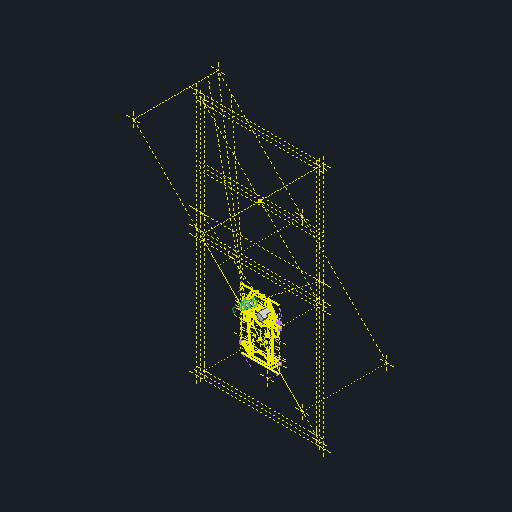
# Autodesk Inventor part: sensormount
Saved by Autodesk Inventor 2023.5 (Build 275446000, 446)
## iProperties
Created: 2025-01-19
Part Number: sensormount
Material: 一般
Document SubType Name: Modeling
Designer: IshiiLabHonda
Density: 1 g/cm^3
Appearance: 既定
Author: IshiiLabHonda
Autodesk Inventor part; units mm, degrees
ref_plane "YZ Plane" through (0, 0, 0) normal (1, 0, 0) x (0, 1, 0)
ref_plane "XZ Plane" through (0, 0, 0) normal (0, 1, 0) x (-1, 0, 0)
ref_plane "XY Plane" through (0, 0, 0) normal (0, 0, 1) x (1, 0, 0)
derived "chassis.ipt"
sketch "スケッチ1" plane through (0, 0, 0) normal (0, 0, 1) x (1, 0, 0)
  line L0 (-90, 90) -> (90, 90) construction
  line L1 (90, 90) -> (90, -90) construction
  line L2 (90, -90) -> (-90, -90) construction
  line L3 (-90, -90) -> (-90, 90) construction
  line L4 (-90, 90) -> (-90, 270) construction
  line L5 (-90, 270) -> (90, 270) construction
  line L6 (90, 270) -> (90, 90) construction
  line L7 (-90, 90) -> (90, -90) construction
  line L8 (90, 90) -> (-90, -90) construction
  line L9 (0, 0) -> (0, 10) construction
  line L10 (0, 0) -> (10, 0) construction
  line L11 (-90, 270) -> (90, 90) construction
  line L12 (-90, 90) -> (90, 270) construction
  line L13 (-96, 276) -> (96, 276) construction
  line L14 (96, 276) -> (96, -96) construction
  line L15 (96, -96) -> (-96, -96) construction
  line L16 (-96, -96) -> (-96, 276) construction
  line L17 (-84, 264) -> (84, 264) construction
  line L18 (84, 264) -> (84, -84) construction
  line L19 (84, -84) -> (-84, -84) construction
  line L20 (-84, -84) -> (-84, 264) construction
  line L21 (-96, 96) -> (96, 96) construction
  line L22 (-96, 84) -> (96, 84) construction
  line L23 (-63.6396, 63.6396) -> (63.6396, 190.9188) construction
  line L24 (63.6396, 190.9188) -> (190.9188, 63.6396) construction
  line L25 (190.9188, 63.6396) -> (63.6396, -63.6396) construction
  line L26 (63.6396, -63.6396) -> (-63.6396, 63.6396) construction
  line L27 (-190.9188, 190.9188) -> (-63.6396, 318.1981) construction
  line L28 (-63.6396, 318.1981) -> (63.6396, 190.9188) construction
  line L29 (-63.6396, 63.6396) -> (-190.9188, 190.9188) construction
  line L30 (-96, 120) -> (96, 120) construction
  line L31 (-96, 186) -> (96, 186) construction
  line L32 (-96, 174) -> (96, 174) construction
  line L33 (-96, 180) -> (96, 180) construction
  point P0 (-63.6396, 318.1981)
  point P1 (-90, 120)
  point P2 (90, 120)
  point P3 (0, 180)
sketch "スケッチ2" plane through (0, 0, 0) normal (0, 0, 1) x (1, 0, 0)
  line L0 (63.6396, 190.9188) -> (190.9188, 63.6396) construction
  line L1 (-63.6396, 318.1981) -> (63.6396, 190.9188) construction
  line L2 (-84, 264) -> (84, 264) construction
  line L3 (-90, 270) -> (90, 270) construction
  line L4 (90, 270) -> (90, 90) construction
  line L5 (-96, 276) -> (96, 276) construction
  line L6 (-90, 90) -> (90, 270) construction
  line L7 (-90, 270) -> (90, 90) construction
  line L8 (-63.6396, 63.6396) -> (63.6396, 190.9188) construction
  line L9 (-96, 120) -> (96, 120) construction
  line L10 (-90, 90) -> (90, 90) construction
  line L11 (-96, 96) -> (96, 96) construction
  line L12 (-96, 84) -> (96, 84) construction
  line L13 (90, -90) -> (-90, -90) construction
  line L14 (0, 0) -> (0, 10) construction
  line L15 (0, 0) -> (10, 0) construction
  line L16 (190.9188, 63.6396) -> (63.6396, -63.6396) construction
  line L17 (63.6396, -63.6396) -> (-63.6396, 63.6396) construction
  line L18 (84, -84) -> (-84, -84) construction
  line L19 (96, -96) -> (-96, -96) construction
  line L20 (-90, 90) -> (-90, 270) construction
  line L21 (-63.6396, 63.6396) -> (-190.9188, 190.9188) construction
  line L22 (-190.9188, 190.9188) -> (-63.6396, 318.1981) construction
  line L23 (96, 276) -> (96, -96) construction
  line L24 (-96, -96) -> (-96, 276) construction
  line L25 (84, 264) -> (84, -84) construction
  line L26 (-84, -84) -> (-84, 264) construction
  line L27 (90, 90) -> (90, -90) construction
  line L28 (-90, 90) -> (90, -90) construction
  line L29 (90, 90) -> (-90, -90) construction
  line L30 (-90, -90) -> (-90, 90) construction
  circle A0 centre (0, 0) radius 16 construction
  circle A1 centre (0, 0) radius 7.5 construction
  line L31 (20, 11.5) -> (28.75, 11.5) construction
  line L32 (28.75, 11.5) -> (28.75, -11.5) construction
  line L33 (28.75, -11.5) -> (20, -11.5) construction
  line L34 (20, -11.5) -> (20, 11.5) construction
  line L35 (20, 11.5) -> (18, 11.5) construction
  line L36 (18, 11.5) -> (18, -11.5) construction
  line L37 (18, -11.5) -> (20, -11.5) construction
  line L38 (18, 1.5) -> (17, 1.5) construction
  line L39 (17, -1.5) -> (18, -1.5) construction
  line L40 (-17, 26) -> (17, 26) construction
  line L41 (17, 26) -> (17, -20) construction
  line L42 (17, -20) -> (-17, -20) construction
  line L43 (-17, -20) -> (-17, 26) construction
  line L44 (-20, 11.5) -> (-18, 11.5) construction
  line L45 (-17, -1.5) -> (-18, -1.5) construction
  line L46 (-20, -11.5) -> (-20, 11.5) construction
  line L47 (-18, 11.5) -> (-18, -11.5) construction
  line L48 (-28.75, -11.5) -> (-20, -11.5) construction
  line L49 (-20, 11.5) -> (-28.75, 11.5) construction
  line L50 (-28.75, 11.5) -> (-28.75, -11.5) construction
  line L51 (-18, -11.5) -> (-20, -11.5) construction
  line L52 (-18, 1.5) -> (-17, 1.5) construction
  line L53 (-14.5, 26) -> (-14.5, -20) construction
  line L54 (14.5, 26) -> (14.5, -20) construction
  line L55 (-10.5, 26) -> (-10.5, 21) construction
  line L56 (-10.5, 21) -> (-14.5, 21) construction
  line L57 (-14.5, 26) -> (-10.5, 21) construction
  line L58 (-10.5, 26) -> (-14.5, 21) construction
  circle A2 centre (-12.5, 23.5) radius 1 construction
  line L59 (10.5, 26) -> (10.5, 21) construction
  line L60 (10.5, 21) -> (14.5, 21) construction
  line L61 (10.5, 26) -> (14.5, 21) construction
  line L62 (10.5, 21) -> (14.5, 26) construction
  circle A3 centre (12.5, 23.5) radius 1 construction
  line L63 (-14.5, -15) -> (-10.5, -15) construction
  line L64 (-10.5, -15) -> (-10.5, -20) construction
  line L65 (10.5, -20) -> (10.5, -15) construction
  line L66 (10.5, -15) -> (14.5, -15) construction
  line L67 (-14.5, -15) -> (-10.5, -20) construction
  line L68 (-10.5, -15) -> (-14.5, -20) construction
  circle A4 centre (-12.5, -17.5) radius 1 construction
  line L69 (10.5, -15) -> (14.5, -20) construction
  line L70 (14.5, -15) -> (10.5, -20) construction
  circle A5 centre (12.5, -17.5) radius 1 construction
  point P0 (90, 120)
  point P1 (-90, 120)
  point P2 (-63.6396, 318.1981)
  point P3 (-12.5, -17.5)
sketch "スケッチ3" plane through (0, 0, 0) normal (0, 0, 1) x (1, 0, 0)
  line L0 (63.6396, 190.9188) -> (190.9188, 63.6396) construction
  line L1 (-63.6396, 318.1981) -> (63.6396, 190.9188) construction
  line L2 (-84, 264) -> (84, 264) construction
  line L3 (-90, 270) -> (90, 270) construction
  line L4 (90, 270) -> (90, 90) construction
  line L5 (-96, 276) -> (96, 276) construction
  line L6 (-90, 90) -> (90, 270) construction
  line L7 (-90, 270) -> (90, 90) construction
  line L8 (-63.6396, 63.6396) -> (63.6396, 190.9188) construction
  line L9 (-96, 120) -> (96, 120) construction
  line L10 (-90, 90) -> (90, 90) construction
  line L11 (-96, 96) -> (96, 96) construction
  line L12 (-96, 84) -> (96, 84) construction
  line L13 (90, -90) -> (-90, -90) construction
  line L14 (0, 0) -> (0, 10) construction
  line L15 (0, 0) -> (10, 0) construction
  line L16 (190.9188, 63.6396) -> (63.6396, -63.6396) construction
  line L17 (63.6396, -63.6396) -> (-63.6396, 63.6396) construction
  line L18 (84, -84) -> (-84, -84) construction
  line L19 (96, -96) -> (-96, -96) construction
  line L20 (-90, 90) -> (-90, 270) construction
  line L21 (-63.6396, 63.6396) -> (-190.9188, 190.9188) construction
  line L22 (-190.9188, 190.9188) -> (-63.6396, 318.1981) construction
  line L23 (96, 276) -> (96, -96) construction
  line L24 (-96, -96) -> (-96, 276) construction
  line L25 (84, 264) -> (84, -84) construction
  line L26 (-84, -84) -> (-84, 264) construction
  line L27 (90, 90) -> (90, -90) construction
  line L28 (-90, 90) -> (90, -90) construction
  line L29 (90, 90) -> (-90, -90) construction
  line L30 (-90, -90) -> (-90, 90) construction
  line L31 (-18, 1.5) -> (-17, 1.5) construction
  line L32 (-17, -1.5) -> (-18, -1.5) construction
  line L33 (-20, 11.5) -> (-18, 11.5) construction
  line L34 (-28.75, 11.5) -> (-28.75, -11.5) construction
  line L35 (63.6396, -63.6396) -> (-63.6396, 63.6396) construction
  line L36 (84, -84) -> (-84, -84) construction
  line L37 (-90, -90) -> (-90, 90) construction
  line L38 (96, -96) -> (-96, -96) construction
  line L39 (-90, 90) -> (90, 90) construction
  line L40 (90, -90) -> (-90, -90) construction
  line L41 (90, 90) -> (-90, -90) construction
  line L42 (-90, 90) -> (90, -90) construction
  line L43 (90, 90) -> (90, -90) construction
  line L44 (-28.75, -11.5) -> (-20, -11.5) construction
  line L45 (-20, 11.5) -> (-28.75, 11.5) construction
  line L46 (-18, 11.5) -> (-18, -11.5) construction
  line L47 (-18, -11.5) -> (-20, -11.5) construction
  line L48 (0, 0) -> (0, 10) construction
  line L49 (0, 0) -> (10, 0) construction
  circle A0 centre (0, 0) radius 16 construction
  circle A1 centre (0, 0) radius 7.5 construction
  line L50 (-14.5, 26) -> (-14.5, -20) construction
  line L51 (-17, 26) -> (17, 26) construction
  line L52 (-17, -20) -> (-17, 26) construction
  line L53 (17, -20) -> (-17, -20) construction
  line L54 (-14.5, -15) -> (-10.5, -15) construction
  circle A2 centre (-12.5, -17.5) radius 1 construction
  line L55 (-10.5, -15) -> (-14.5, -20) construction
  line L56 (-14.5, -15) -> (-10.5, -20) construction
  line L57 (-63.6396, 318.1981) -> (63.6396, 190.9188) construction
  line L58 (-84, 264) -> (84, 264) construction
  line L59 (-90, 270) -> (90, 270) construction
  line L60 (90, 270) -> (90, 90) construction
  line L61 (-96, 276) -> (96, 276) construction
  line L62 (-90, 90) -> (90, 270) construction
  line L63 (-90, 270) -> (90, 90) construction
  line L64 (-63.6396, 63.6396) -> (63.6396, 190.9188) construction
  line L65 (-96, 120) -> (96, 120) construction
  line L66 (-96, 96) -> (96, 96) construction
  line L67 (-96, 84) -> (96, 84) construction
  line L68 (84, 264) -> (84, -84) construction
  line L69 (96, 276) -> (96, -96) construction
  line L70 (-96, -96) -> (-96, 276) construction
  line L71 (-84, -84) -> (-84, 264) construction
  line L72 (-63.6396, 63.6396) -> (-190.9188, 190.9188) construction
  line L73 (-90, 90) -> (-90, 270) construction
  line L74 (-190.9188, 190.9188) -> (-63.6396, 318.1981) construction
  line L75 (-20, -11.5) -> (-20, 11.5) construction
  line L76 (10.5, -15) -> (14.5, -15) construction
  line L77 (10.5, -20) -> (10.5, -15) construction
  circle A3 centre (12.5, -17.5) radius 1 construction
  line L78 (10.5, -15) -> (14.5, -20) construction
  line L79 (14.5, -15) -> (10.5, -20) construction
  line L80 (-10.5, -15) -> (-10.5, -20) construction
  line L81 (63.6396, 190.9188) -> (190.9188, 63.6396) construction
  line L82 (190.9188, 63.6396) -> (63.6396, -63.6396) construction
  line L83 (20, 11.5) -> (28.75, 11.5) construction
  line L84 (28.75, 11.5) -> (28.75, -11.5) construction
  line L85 (17, -1.5) -> (18, -1.5) construction
  line L86 (18, -11.5) -> (20, -11.5) construction
  line L87 (28.75, -11.5) -> (20, -11.5) construction
  line L88 (14.5, 26) -> (14.5, -20) construction
  line L89 (17, 26) -> (17, -20) construction
  line L90 (18, 11.5) -> (18, -11.5) construction
  line L91 (20, -11.5) -> (20, 11.5) construction
  line L92 (20, 11.5) -> (18, 11.5) construction
  line L93 (18, 1.5) -> (17, 1.5) construction
  line L94 (-10.5, 26) -> (-10.5, 21) construction
  line L95 (10.5, 21) -> (14.5, 21) construction
  circle A4 centre (12.5, 23.5) radius 1 construction
  line L96 (10.5, 26) -> (14.5, 21) construction
  line L97 (10.5, 21) -> (14.5, 26) construction
  line L98 (10.5, 26) -> (10.5, 21) construction
  line L99 (-10.5, 21) -> (-14.5, 21) construction
  circle A5 centre (-12.5, 23.5) radius 1 construction
  line L100 (-14.5, 26) -> (-10.5, 21) construction
  line L101 (-10.5, 26) -> (-14.5, 21) construction
  line L102 (-33.2155, 41.4468) -> (33.2155, 41.4468) construction
  line L103 (29.25, 58) -> (29.25, -32) construction
  line L104 (29.25, -32) -> (-29.25, -32) construction
  line L105 (-29.25, -32) -> (-29.25, 58) construction
  line L106 (-29.25, 8.5) -> (-17, 8.5) construction
  line L107 (-17, 8.5) -> (-17, -8.5) construction
  line L108 (-17, -8.5) -> (-29.25, -8.5) construction
  line L109 (29.25, 8.5) -> (17, 8.5) construction
  line L110 (17, 8.5) -> (17, -8.5) construction
  line L111 (17, -8.5) -> (29.25, -8.5) construction
  line L112 (-20.1078, 31.6026) -> (-18.8984, 22.9366) construction
  line L113 (7.9335, 41.7018) -> (10.9773, 45.6686) construction
  line L114 (6.7297, 41.365) -> (10.991, 46.9185) construction
  line L115 (11.8865, 37.4081) -> (6.7297, 41.365) construction
  line L116 (10.991, 46.9185) -> (11.8865, 37.4081) construction
  line L117 (11.9003, 38.658) -> (10.9773, 45.6686) construction
  line L118 (11.9003, 38.658) -> (7.9335, 41.7018) construction
  line L119 (11.8865, 37.4081) -> (14.2666, 35.5818) construction
  line L120 (10.9773, 45.6686) -> (14.9441, 42.6248) construction
  line L121 (7.9335, 41.7018) -> (14.9441, 42.6248) construction
  line L122 (14.9441, 42.6248) -> (11.9003, 38.658) construction
  line L123 (6.7297, 41.365) -> (16.1478, 42.9616) construction
  line L124 (10.991, 46.9185) -> (16.1478, 42.9616) construction
  line L125 (16.1478, 42.9616) -> (11.8865, 37.4081) construction
  line L126 (14.2666, 35.5818) -> (18.5279, 41.1353) construction
  line L127 (18.5279, 41.1353) -> (16.1478, 42.9616) construction
  line L128 (-20.9946, 30.7216) -> (-20.3034, 25.7696) construction
  line L129 (-25.9466, 30.0304) -> (-20.3034, 25.7696) construction
  line L130 (-25.2554, 25.0784) -> (-20.9946, 30.7216) construction
  line L131 (-27.0406, 30.635) -> (-20.1078, 31.6026) construction
  line L132 (-25.2554, 25.0784) -> (-25.9466, 30.0304) construction
  line L133 (-18.8984, 22.9366) -> (-25.8312, 21.969) construction
  line L134 (-25.8312, 21.969) -> (-27.0406, 30.635) construction
  line L135 (-63.6396, 318.1981) -> (-23.125, 27.9) construction
  line L136 (11.4388, 42.1633) -> (-90, 120) construction
  line L137 (-23.125, 27.9) -> (-78.8228, 303.0149) construction
  line L138 (-23.125, 27.9) -> (-44.1788, 298.7372) construction
  line L139 (-11.4388, 42.1633) -> (90, 120) construction
  line L140 (-10.9773, 45.6686) -> (-7.9335, 41.7018) construction
  line L141 (-10.991, 46.9185) -> (-6.7297, 41.365) construction
  line L142 (-16.1478, 42.9616) -> (-10.991, 46.9185) construction
  line L143 (-6.7297, 41.365) -> (-16.1478, 42.9616) construction
  line L144 (-14.9441, 42.6248) -> (-7.9335, 41.7018) construction
  line L145 (-14.9441, 42.6248) -> (-10.9773, 45.6686) construction
  line L146 (-16.1478, 42.9616) -> (-18.5279, 41.1353) construction
  line L147 (-7.9335, 41.7018) -> (-11.9003, 38.658) construction
  line L148 (-10.9773, 45.6686) -> (-11.9003, 38.658) construction
  line L149 (-10.991, 46.9185) -> (-11.8865, 37.4081) construction
  line L150 (-6.7297, 41.365) -> (-11.8865, 37.4081) construction
  line L151 (-11.8865, 37.4081) -> (-16.1478, 42.9616) construction
  line L152 (-18.5279, 41.1353) -> (-14.2666, 35.5818) construction
  line L153 (-14.2666, 35.5818) -> (-11.8865, 37.4081) construction
  line L154 (-11.9003, 38.658) -> (-14.9441, 42.6248) construction
  line L155 (-33.2155, 41.4468) -> (-29.25, 58) construction
  line L156 (33.2155, 41.4468) -> (29.25, 58) construction
  line L157 (-29.25, -32) -> (-13.618, -44.2445) construction
  line L158 (11.1121, -46.2074) -> (29.25, -32) construction
  circle A6 centre (-8.395, 38.1965) radius 0.625 construction
  circle A7 centre (-8.395, 38.1965) radius 0.8 construction
  circle A8 centre (-8.395, 38.1965) radius 1.5 construction
  circle A9 centre (-15.2072, 39.2717) radius 1.5 construction
  circle A10 centre (-15.2072, 39.2717) radius 0.8 construction
  circle A11 centre (-15.2072, 39.2717) radius 0.625 construction
  line L159 (-25.9466, 30.0304) -> (-26.1449, 30.0022) construction
  line L160 (-20.3034, 25.7696) -> (-25.2554, 25.0784) construction
  line L161 (-26.1422, 24.1974) -> (-19.2094, 25.165) construction
  line L162 (-25.601, 27.5544) -> (-20.649, 28.2456) construction
  line L163 (-22.3648, 22.4528) -> (-22.7794, 25.424) construction
  circle A12 centre (-18.173, 28.5911) radius 0.625 construction
  circle A13 centre (-18.173, 28.5911) radius 0.8
  circle A14 centre (-18.173, 28.5911) radius 1.5 construction
  circle A15 centre (-27.1405, 25.3286) radius 0.625 construction
  circle A16 centre (-27.1405, 25.3286) radius 0.8
  line L164 (-25.9466, 30.0304) -> (-20.9946, 30.7216) construction
  circle A17 centre (18.173, 28.5911) radius 0.625 construction
  circle A18 centre (18.173, 28.5911) radius 0.8
  circle A19 centre (18.173, 28.5911) radius 1.5 construction
  circle A20 centre (27.1405, 25.3286) radius 0.625 construction
  circle A21 centre (27.1405, 25.3286) radius 0.8
  circle A22 centre (27.1405, 25.3286) radius 1.5 construction
  circle A23 centre (15.2072, 39.2717) radius 1.5 construction
  circle A24 centre (15.2072, 39.2717) radius 0.625 construction
  circle A25 centre (15.2072, 39.2717) radius 0.8
  circle A26 centre (8.395, 38.1965) radius 1.5 construction
  circle A27 centre (8.395, 38.1965) radius 0.8
  circle A28 centre (8.395, 38.1965) radius 0.625 construction
  line L165 (-29.25, -32) -> (29.25, -32)
  line L166 (-29.25, 58) -> (29.25, 58)
  line L167 (-11.4388, 42.1633) -> (-8.395, 38.1965) construction
  line L168 (-29.25, 28.2016) -> (-12.0459, 58)
  line L169 (-29.25, -17.6878) -> (-14.9378, -32)
  line L170 (29.25, 28.2016) -> (12.0459, 58)
  line L171 (29.25, -17.6878) -> (14.9378, -32)
  line L172 (-9.7365, 54) -> (9.7365, 54)
  line L173 (9.7365, 54) -> (25.25, 27.1298)
  line L174 (25.25, 27.1298) -> (25.25, 14.5)
  line L175 (25.25, 14.5) -> (17, 14.5)
  line L176 (3.695, 18.0905) -> (-3.695, 18.0905)
  line L177 (-17, 14.5) -> (-25.25, 14.5)
  line L178 (-25.25, 14.5) -> (-25.25, 27.1298)
  line L179 (-25.25, 27.1298) -> (-9.7365, 54)
  line L180 (18.8984, 22.9366) -> (25.8312, 21.969) construction
  line L181 (25.8312, 21.969) -> (27.0406, 30.635) construction
  line L182 (20.1078, 31.6026) -> (18.8984, 22.9366) construction
  line L183 (20.3034, 25.7696) -> (25.2554, 25.0784) construction
  line L184 (26.1422, 24.1974) -> (19.2094, 25.165) construction
  line L185 (25.9466, 30.0304) -> (20.3034, 25.7696) construction
  line L186 (25.2554, 25.0784) -> (20.9946, 30.7216) construction
  line L187 (20.9946, 30.7216) -> (20.3034, 25.7696) construction
  line L188 (25.9466, 30.0304) -> (20.9946, 30.7216) construction
  line L189 (25.2554, 25.0784) -> (25.9466, 30.0304) construction
  line L190 (27.0406, 30.635) -> (20.1078, 31.6026) construction
  line L191 (-9.7365, 22.9366) -> (-9.7365, 26)
  line L192 (9.7365, 22.9366) -> (9.7365, 26)
  line L193 (9.7365, 26) -> (17, 26)
  line L194 (17, 26) -> (17, 14.5)
  line L195 (-9.7365, 26) -> (-17, 26)
  line L196 (-17, 26) -> (-17, 14.5)
  line L197 (-9.7365, 22.9366) -> (-3.695, 18.0905)
  line L198 (9.7365, 22.9366) -> (3.695, 18.0905)
  line L199 (-17, -14.5) -> (-25.25, -14.5)
  line L200 (-25.25, -14.5) -> (-25.25, -16.0309)
  line L201 (-25.25, -16.0309) -> (-13.2809, -28)
  line L202 (-13.2809, -28) -> (13.2809, -28)
  line L203 (13.2809, -28) -> (25.25, -16.0309)
  line L204 (25.25, -16.0309) -> (25.25, -14.5)
  line L205 (25.25, -14.5) -> (17, -14.5)
  line L206 (17, -14.5) -> (17, -20.8804)
  line L207 (17, -20.8804) -> (6.6466, -20.8804)
  line L208 (6.6466, -20.8804) -> (4.7017, -18.0332)
  line L209 (4.7017, -18.0332) -> (-4.7017, -18.0332)
  line L210 (-4.7017, -18.0332) -> (-6.6466, -20.8804)
  line L211 (-6.6466, -20.8804) -> (-17, -20.8804)
  line L212 (-17, -20.8804) -> (-17, -14.5)
  line L213 (-16.1661, 42.8636) -> (16.1661, 42.8636)
  line L214 (-20.6579, 35.0836) -> (20.6579, 35.0836)
  line L215 (-22.045, 32.6811) -> (-12.2942, 28.5594)
  line L216 (-12.2942, 28.5594) -> (12.2942, 28.5594)
  line L217 (12.2942, 28.5594) -> (22.045, 32.6811)
  line L218 (-25.25, 25.1515) -> (25.25, 25.1515)
  circle A29 centre (-27.1405, 25.3286) radius 1.5 construction
  line L219 (-7.5571, 35.0836) -> (-5.0762, 37.1727)
  line L220 (-5.0762, 37.1727) -> (5.0762, 37.1727)
  line L221 (5.0762, 37.1727) -> (7.5571, 35.0836)
  line L222 (0, 41.1322) -> (6.2476, 42.8636)
  line L223 (-6.2476, 42.8636) -> (0, 41.1322)
  line L224 (-17, 18.9574) -> (-20.6579, 14.5)
  line L225 (17, 18.9574) -> (20.6579, 14.5)
  point P0 (29.25, 35.054)
  point P1 (-20.75, 28.7194)
  point P2 (-26.5183, 35.054)
  point P3 (-29.25, 26.6905)
  point P4 (26.5183, 35.054)
  point P5 (29.25, 26.6905)
  point P6 (-29.25, -18.5)
  point P7 (29.25, -18.5)
  point P8 (16.5079, 42.2717)
  point P9 (-4.3925, 58)
  point P10 (4.5158, 58)
sketch "スケッチ4" plane through (0, 0, 0) normal (0, 0, 1) x (1, 0, 0)
  line L0 (0, 0) -> (0, 10) construction
  line L1 (0, 0) -> (10, 0) construction
  line L2 (-18, 1.5) -> (-17, 1.5) construction
  line L3 (-20, 11.5) -> (-28.75, 11.5) construction
  line L4 (-17, -1.5) -> (-18, -1.5) construction
  line L5 (-18, 11.5) -> (-18, -11.5) construction
  line L6 (-18, -11.5) -> (-20, -11.5) construction
  line L7 (-20, -11.5) -> (-20, 11.5) construction
  line L8 (-28.75, -11.5) -> (-20, -11.5) construction
  line L9 (-28.75, 11.5) -> (-28.75, -11.5) construction
  line L10 (20, 11.5) -> (28.75, 11.5) construction
  line L11 (28.75, 11.5) -> (28.75, -11.5) construction
  line L12 (28.75, -11.5) -> (20, -11.5) construction
  line L13 (18, -11.5) -> (20, -11.5) construction
  line L14 (17, -1.5) -> (18, -1.5) construction
  line L15 (18, 1.5) -> (17, 1.5) construction
  line L16 (20, -11.5) -> (20, 11.5) construction
  line L17 (20, 11.5) -> (18, 11.5) construction
  line L18 (18, 11.5) -> (18, -11.5) construction
  circle A0 centre (0, 0) radius 7.5 construction
  line L19 (17, -20) -> (-17, -20) construction
  circle A1 centre (0, 0) radius 16 construction
  line L20 (14.5, 26) -> (14.5, -20) construction
  line L21 (-17, 26) -> (17, 26) construction
  line L22 (-14.5, 26) -> (-14.5, -20) construction
  line L23 (-17, -20) -> (-17, 26) construction
  line L24 (17, 26) -> (17, -20) construction
  line L25 (-20, 11.5) -> (-18, 11.5) construction
  line L26 (-10.5, 21) -> (-14.5, 21) construction
  line L27 (-10.5, 26) -> (-10.5, 21) construction
  circle A2 centre (-12.5, 23.5) radius 1 construction
  line L28 (-10.5, 26) -> (-14.5, 21) construction
  line L29 (-14.5, 26) -> (-10.5, 21) construction
  line L30 (10.5, 21) -> (14.5, 21) construction
  line L31 (10.5, 26) -> (10.5, 21) construction
  circle A3 centre (12.5, 23.5) radius 1 construction
  line L32 (10.5, 26) -> (14.5, 21) construction
  line L33 (10.5, 21) -> (14.5, 26) construction
  line L34 (-14.5, -15) -> (-10.5, -15) construction
  circle A4 centre (-12.5, -17.5) radius 1 construction
  line L35 (-14.5, -15) -> (-10.5, -20) construction
  line L36 (-10.5, -15) -> (-14.5, -20) construction
  line L37 (-10.5, -15) -> (-10.5, -20) construction
  line L38 (10.5, -15) -> (14.5, -15) construction
  line L39 (10.5, -20) -> (10.5, -15) construction
  circle A5 centre (12.5, -17.5) radius 1 construction
  line L40 (10.5, -15) -> (14.5, -20) construction
  line L41 (14.5, -15) -> (10.5, -20) construction
  line L42 (0, 0) -> (0, 10) construction
  line L43 (0, 0) -> (10, 0) construction
  line L44 (0, 0) -> (0, 10) construction
  line L45 (0, 0) -> (10, 0) construction
  line L46 (-18, 1.5) -> (-17, 1.5) construction
  line L47 (-17, -1.5) -> (-18, -1.5) construction
  line L48 (-20, 11.5) -> (-18, 11.5) construction
  line L49 (-28.75, 11.5) -> (-28.75, -11.5) construction
  line L50 (-33.2155, 41.4468) -> (33.2155, 41.4468) construction
  line L51 (-20, 11.5) -> (-28.75, 11.5) construction
  line L52 (-17, 26) -> (17, 26) construction
  line L53 (-10.5, 21) -> (-14.5, 21) construction
  line L54 (-10.5, 26) -> (-10.5, 21) construction
  line L55 (-14.5, 26) -> (-10.5, 21) construction
  line L56 (10.5, 21) -> (14.5, 21) construction
  line L57 (10.5, 26) -> (14.5, 21) construction
  line L58 (20, 11.5) -> (28.75, 11.5) construction
  line L59 (20, 11.5) -> (18, 11.5) construction
  line L60 (0, 0) -> (0, 10) construction
  line L61 (-28.75, -11.5) -> (-20, -11.5) construction
  line L62 (-29.25, -32) -> (-29.25, 58) construction
  line L63 (29.25, 35.054) -> (29.25, -32) construction
  line L64 (28.75, 11.5) -> (28.75, -11.5) construction
  circle A6 centre (0, 0) radius 7.5 construction
  line L65 (-18, -11.5) -> (-20, -11.5) construction
  line L66 (20, -11.5) -> (20, 11.5) construction
  line L67 (18, 11.5) -> (18, -11.5) construction
  circle A7 centre (0, 0) radius 16 construction
  line L68 (17, 26) -> (17, -20) construction
  line L69 (14.5, 26) -> (14.5, -20) construction
  line L70 (-17, -20) -> (-17, 26) construction
  line L71 (-14.5, 26) -> (-14.5, -20) construction
  line L72 (-18, 11.5) -> (-18, -11.5) construction
  line L73 (-10.5, 26) -> (-14.5, 21) construction
  line L74 (0, 0) -> (10, 0) construction
  line L75 (10.5, -15) -> (14.5, -15) construction
  line L76 (29.25, -32) -> (-29.25, -32) construction
  line L77 (17, -20) -> (-17, -20) construction
  circle A8 centre (12.5, -17.5) radius 1 construction
  line L78 (14.5, -15) -> (10.5, -20) construction
  line L79 (10.5, -15) -> (14.5, -20) construction
  line L80 (10.5, -20) -> (10.5, -15) construction
  circle A9 centre (-12.5, -17.5) radius 1 construction
  line L81 (-10.5, -15) -> (-14.5, -20) construction
  line L82 (-14.5, -15) -> (-10.5, -20) construction
  line L83 (-10.5, -15) -> (-10.5, -20) construction
  line L84 (-14.5, -15) -> (-10.5, -15) construction
  line L85 (-27.0406, 30.635) -> (-20.1078, 31.6026) construction
  line L86 (-20.9946, 30.7216) -> (-20.3034, 25.7696) construction
  line L87 (-25.9466, 30.0304) -> (-20.3034, 25.7696) construction
  circle A10 centre (-12.5, 23.5) radius 1 construction
  line L88 (17, -1.5) -> (18, -1.5) construction
  line L89 (18, -11.5) -> (20, -11.5) construction
  line L90 (18, 1.5) -> (17, 1.5) construction
  line L91 (17, 8.5) -> (17, -8.5) construction
  line L92 (29.25, 8.5) -> (17, 8.5) construction
  line L93 (28.75, -11.5) -> (20, -11.5) construction
  line L94 (17, -8.5) -> (29.25, -8.5) construction
  line L95 (-17, 8.5) -> (-17, -8.5) construction
  line L96 (-17, -8.5) -> (-29.25, -8.5) construction
  line L97 (-29.25, 8.5) -> (-17, 8.5) construction
  line L98 (-20, -11.5) -> (-20, 11.5) construction
  line L99 (-29.25, -32) -> (-13.618, -44.2445) construction
  line L100 (10.5, 26) -> (10.5, 21) construction
  line L101 (10.5, 21) -> (14.5, 26) construction
  line L102 (11.1121, -46.2074) -> (29.25, -32) construction
  circle A11 centre (12.5, 23.5) radius 1 construction
  line L103 (10.991, 46.9185) -> (16.1478, 42.9616) construction
  line L104 (11.8865, 37.4081) -> (14.2666, 35.5818) construction
  line L105 (14.2666, 35.5818) -> (18.5279, 41.1353) construction
  line L106 (11.9003, 38.658) -> (10.9773, 45.6686) construction
  line L107 (18.5279, 41.1353) -> (16.1478, 42.9616) construction
  line L108 (7.9335, 41.7018) -> (10.9773, 45.6686) construction
  line L109 (6.7297, 41.365) -> (10.991, 46.9185) construction
  line L110 (11.8865, 37.4081) -> (6.7297, 41.365) construction
  line L111 (10.991, 46.9185) -> (11.8865, 37.4081) construction
  line L112 (10.9773, 45.6686) -> (14.9441, 42.6248) construction
  line L113 (7.9335, 41.7018) -> (14.9441, 42.6248) construction
  line L114 (14.9441, 42.6248) -> (11.9003, 38.658) construction
  line L115 (16.1478, 42.9616) -> (11.8865, 37.4081) construction
  line L116 (6.7297, 41.365) -> (16.1478, 42.9616) construction
  line L117 (33.2155, 41.4468) -> (29.25, 58) construction
  line L118 (11.9003, 38.658) -> (7.9335, 41.7018) construction
  circle A12 centre (-15.2072, 39.2717) radius 0.8 construction
  circle A13 centre (-15.2072, 39.2717) radius 1.5 projected
  line L119 (-14.2666, 35.5818) -> (-11.8865, 37.4081) construction
  line L120 (-18.5279, 41.1353) -> (-14.2666, 35.5818) construction
  circle A14 centre (-15.2072, 39.2717) radius 0.625 projected
  line L121 (-16.1478, 42.9616) -> (-18.5279, 41.1353) construction
  line L122 (-10.9773, 45.6686) -> (-7.9335, 41.7018) construction
  line L123 (-10.991, 46.9185) -> (-6.7297, 41.365) projected
  line L124 (-11.9003, 38.658) -> (-14.9441, 42.6248) construction
  line L125 (-11.8865, 37.4081) -> (-16.1478, 42.9616) projected
  line L126 (-14.9441, 42.6248) -> (-10.9773, 45.6686) construction
  line L127 (-10.9773, 45.6686) -> (-11.9003, 38.658) construction
  line L128 (-16.1478, 42.9616) -> (-10.991, 46.9185) projected
  line L129 (-10.991, 46.9185) -> (-11.8865, 37.4081) construction
  line L130 (-14.9441, 42.6248) -> (-7.9335, 41.7018) construction
  line L131 (-6.7297, 41.365) -> (-16.1478, 42.9616) construction
  circle A15 centre (-8.395, 38.1965) radius 0.625 projected
  circle A16 centre (-8.395, 38.1965) radius 0.8 construction
  circle A17 centre (-8.395, 38.1965) radius 1.5 projected
  line L132 (-6.7297, 41.365) -> (-11.8865, 37.4081) projected
  line L133 (-7.9335, 41.7018) -> (-11.9003, 38.658) construction
  line L134 (-25.2554, 25.0784) -> (-25.9466, 30.0304) construction
  line L135 (-20.1078, 31.6026) -> (-18.8984, 22.9366) construction
  line L136 (-25.2554, 25.0784) -> (-20.9946, 30.7216) construction
  line L137 (-18.8984, 22.9366) -> (-25.8312, 21.969) construction
  line L138 (-25.8312, 21.969) -> (-27.0406, 30.635) construction
  line L139 (-33.2155, 41.4468) -> (-29.25, 58) construction
  line L140 (-25.9466, 30.0304) -> (-26.1449, 30.0022) construction
  line L141 (-22.3648, 22.4528) -> (-22.7794, 25.424) construction
  line L142 (-25.601, 27.5544) -> (-20.649, 28.2456) construction
  line L143 (-20.3034, 25.7696) -> (-25.2554, 25.0784) construction
  line L144 (-26.1422, 24.1974) -> (-19.2094, 25.165) construction
  circle A18 centre (8.395, 38.1965) radius 0.625 construction
  circle A19 centre (8.395, 38.1965) radius 0.8 projected
  circle A20 centre (8.395, 38.1965) radius 1.5 projected
  circle A21 centre (15.2072, 39.2717) radius 0.8 projected
  circle A22 centre (15.2072, 39.2717) radius 1.5 projected
  circle A23 centre (15.2072, 39.2717) radius 0.625 construction
  point P0 (-12.5, -17.5)
  point P1 (-20.75, 28.7194)
  point P2 (-23.125, 27.9)
  point P3 (11.4388, 42.1633)
  point P4 (-29.25, -18.5)
  point P5 (-13.618, -44.2445)
  point P6 (29.25, -18.5)
  point P7 (26.5183, 35.054)
  point P8 (29.25, 26.6905)
  point P9 (-11.4388, 42.1633)
  point P10 (-26.5183, 35.054)
  point P11 (-29.25, 26.6905)
  point P12 (-23.125, 27.9)
  point P13 (29.25, 58)
  constraints: 25 other
extrude "押し出し1" add sketch "スケッチ4" along normal blind 13.5 contours L125 L128 L123 L132
ref_plane "作業平面1" through (-11.8865, 37.4081, 0) normal (-0.7933533, -0.6087614, 0) x (0, 0, 1)
sketch "スケッチ5" plane through (-11.8865, 37.4081, 0) normal (-0.7933533, -0.6087614, 0) x (0, 0, 1)
  line L0 (0, 7) -> (0, 0) projected
  line L1 (0, 0) -> (13.5, 0) projected
  line L2 (13.5, 7) -> (13.5, 0) projected
  line L3 (0, 7) -> (13.5, 7) projected
  circle A0 centre (10, 3.5) radius 2.5
  circle A1 centre (4, 3.5) radius 2.5
  line L4 (13.5, 7) -> (13.5, 0) projected
  line L5 (0, 7) -> (0, 0) projected
  line L6 (13.5, 7) -> (0, 0) construction
  line L7 (0, 7) -> (13.5, 0) construction
  line L8 (13.5, 3.5) -> (0, 3.5) construction
  line L9 (7.5, 7) -> (7.5, 0) construction
  line L10 (6.5, 7) -> (6.5, 0) construction
  line L11 (0, 7) -> (13.5, 7) projected
  line L12 (0, 0) -> (13.5, 0) projected
  line L13 (1.5, 7) -> (1.5, 0) construction
  line L14 (12.5, 7) -> (12.5, 0) construction
  line L15 (6.5, 7) -> (1.5, 0) construction
  line L16 (6.5, 0) -> (1.5, 7) construction
  line L17 (7.5, 7) -> (12.5, 0) construction
  line L18 (7.5, 0) -> (12.5, 7) construction
  line L19 (7, 7) -> (7, 0)
  point P0 (0, -36.9139)
  point P1 (6.75, 3.5)
  point P2 (6.75, 3.5)
  dimension "d4" = 5
  dimension "d5" = 5
  dimension "d6" = 1
  dimension "d7" = 1.5
  dimension "d8" = 1
  constraints: 24 end point, 10 point on line, 7 midpoint, 3 perpendicular, 2 centre point, 2 coincident, 2 parallel, 1 tangent, 1 other
  measures "d4" diameter of A0
  measures "d5" diameter of A1
  measures "d6" distance between parallel lines of L10 L9
  measures "d7" distance between parallel lines of L0 L13
  measures "d8" distance between parallel lines of L14 L2
extrude "押し出し3" cut sketch "スケッチ5" along normal mid plane 20 contours A0 | A1
extrude "押し出し5" add sketch "スケッチ5" along normal blind 3 contours L3 L2 L1 L19
extrude "押し出し4" add sketch "スケッチ4" along normal blind 1 contours A13 | A17
mirror "ミラー1" about plane through (0, 0, 0) normal (1, 0, 0) of "押し出し5", "押し出し3", "押し出し1"
extrude "押し出し6" add sketch "スケッチ4" along normal blind 1 contours A20 | A22
